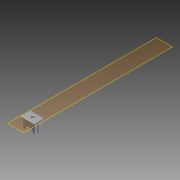
# Autodesk Inventor part: InternalKey
Saved by Autodesk Inventor 2012 (Build 160160000, 160)
## iProperties
Created: 2011-09-20
Part Number: InternalKey
Material: Default
Document SubType Name: Modeling
Designer: KuttaA
Density: 1 g/cm^3
Mass: 2.21175 g
Surface Area: 14.0837 cm^2
Volume: 2.21175 cm^3
Author: KuttaA
Autodesk Inventor part; units mm, degrees
ref_plane "YZ Plane" through (0, 0, 0) normal (1, 0, 0) x (0, 1, 0)
ref_plane "XZ Plane" through (0, 0, 0) normal (0, 1, 0) x (-1, 0, 0)
ref_plane "Work Plane8" through (7.15, 0.8, 25.4) normal (0, 1, 0) x (1, 0, 0)
sketch "Sketch21" plane through (7.15, 0.8, 25.4) normal (0, 1, 0) x (1, 0, 0)
  line L0 (-3, 3) -> (-24, 3)
  line L1 (-3, 197) -> (-3, 3)
  line L2 (-24, 197) -> (-3, 197)
  line L3 (-24, 3) -> (-24, 197)
  line L4 (-4.819988, 19.366667) -> (-3.319988, 19.366667)
  line L5 (-3.319988, 19.366667) -> (-3.319988, 16.033333)
  line L6 (-3.319988, 16.033333) -> (-4.819988, 16.033333)
  line L7 (-4.819988, 16.033333) -> (-4.819988, 12.7)
  line L8 (-4.819988, 12.7) -> (-22.180012, 12.7)
  line L9 (-22.180012, 12.7) -> (-22.180012, 16.033333)
  line L10 (-22.180012, 16.033333) -> (-23.680012, 16.033333)
  line L11 (-23.680012, 16.033333) -> (-23.680012, 19.366667)
  line L12 (-23.680012, 19.366667) -> (-22.180012, 19.366667)
  line L13 (-22.180012, 19.366667) -> (-22.180012, 22.7)
  line L14 (-22.180012, 22.7) -> (-4.819988, 22.7)
  line L15 (-4.819988, 22.7) -> (-4.819988, 19.366667)
  line L16 (-21.880012, 22.4) -> (-21.880012, 19.066667)
  line L17 (-21.880012, 19.066667) -> (-23.380012, 19.066667)
  line L18 (-23.380012, 19.066667) -> (-23.380012, 16.333333)
  line L19 (-23.380012, 16.333333) -> (-21.880012, 16.333333)
  line L20 (-21.880012, 16.333333) -> (-21.880012, 13)
  line L21 (-21.880012, 13) -> (-5.119988, 13)
  line L22 (-5.119988, 13) -> (-5.119988, 16.333333)
  line L23 (-5.119988, 16.333333) -> (-3.619988, 16.333333)
  line L24 (-3.619988, 16.333333) -> (-3.619988, 19.066667)
  line L25 (-3.619988, 19.066667) -> (-5.119988, 19.066667)
  line L26 (-5.119988, 19.066667) -> (-5.119988, 22.4)
  line L27 (-5.119988, 22.4) -> (-21.880012, 22.4)
  point P0 (-7.15, 25.4)
  dimension "d99" = 0.3
  dimension "d100" = 0.3
  dimension "d101" = 0.3
  dimension "d102" = 0.3
  dimension "d103" = 0.3
  dimension "d104" = 0.3
  dimension "d105" = 0.3
  dimension "d106" = 0.3
  dimension "d107" = 0.3
  dimension "d108" = 0.3
  dimension "d109" = 0.3
  dimension "d110" = 0.3
  constraints: 24 end point, 8 parallel, 2 collinear, 2 perpendicular
  measures "d99" distance between parallel lines of L14 L27
  measures "d100" distance between parallel lines of L15 L26
  measures "d101" distance between parallel lines of L4 L25
  measures "d102" distance between parallel lines of L5 L24
  measures "d103" distance between parallel lines of L6 L23
  measures "d104" distance between parallel lines of L7 L22
  measures "d105" distance between parallel lines of L8 L21
  measures "d106" distance between parallel lines of L9 L20
  measures "d107" distance between parallel lines of L10 L19
  measures "d108" distance between parallel lines of L11 L18
  measures "d109" distance between parallel lines of L12 L17
  measures "d110" distance between parallel lines of L13 L16
ref_plane "Work Plane9" through (-1.05, -12.7, 2.7) normal (0, 1, 0) x (0, 0, 1)
sketch "Sketch21 outline for Extrusion20" plane through (7.15, 0.8, 25.4) normal (0, 1, 0) x (1, 0, 0)
  line L0 (-5.119988, 22.4) -> (-21.880012, 22.4)
  line L1 (-5.119988, 19.066667) -> (-5.119988, 22.4)
  line L2 (-3.619988, 19.066667) -> (-5.119988, 19.066667)
  line L3 (-3.619988, 16.333333) -> (-3.619988, 19.066667)
  line L4 (-5.119988, 16.333333) -> (-3.619988, 16.333333)
  line L5 (-5.119988, 13) -> (-5.119988, 16.333333)
  line L6 (-21.880012, 13) -> (-5.119988, 13)
  line L7 (-21.880012, 16.333333) -> (-21.880012, 13)
  line L8 (-23.380012, 16.333333) -> (-21.880012, 16.333333)
  line L9 (-23.380012, 19.066667) -> (-23.380012, 16.333333)
  line L10 (-21.880012, 19.066667) -> (-23.380012, 19.066667)
  line L11 (-21.880012, 22.4) -> (-21.880012, 19.066667)
extrude "Extrusion20" add sketch "Sketch21 outline for Extrusion20" against normal up to surface (13.5 mm away)
sketch "Sketch22" plane through (-14.730012, 0.8, 12.4) normal (0, 0, 1) x (1, 0, 0)
  circle A0 centre (8.380012, -13.5) radius 5 construction
  arc A1 (3.080012, -13.5) -> (13.680012, -13.5) centre (8.380012, -13.5) ccw
  arc A2 (13.680012, -13.5) -> (3.080012, -13.5) centre (8.380012, -13.5) ccw
  point P0 (14.730012, -0.8)
  constraints: 2 point on circle, 1 centre point, 1 concentric
sketch "Sketch22 outline for Extrusion21" plane through (-14.730012, 0.8, 12.4) normal (0, 0, 1) x (1, 0, 0)
  arc A0 (13.680012, -13.5) -> (3.080012, -13.5) centre (8.380012, -13.5) ccw
  arc A1 (3.080012, -13.5) -> (13.680012, -13.5) centre (8.380012, -13.5) ccw
extrude "Extrusion21" cut sketch "Sketch22 outline for Extrusion21" against normal through all
sketch "Sketch23" plane through (7.15, 0.8, 25.4) normal (0, 1, 0) x (1, 0, 0)
  line L0 (-21.880012, 22.4) -> (-21.880012, 19.066667)
  line L1 (-21.880012, 19.066667) -> (-23.380012, 19.066667)
  line L2 (-23.380012, 19.066667) -> (-23.380012, 16.333333)
  line L3 (-23.380012, 16.333333) -> (-21.880012, 16.333333)
  line L4 (-21.880012, 16.333333) -> (-21.880012, 13)
  line L5 (-21.880012, 13) -> (-5.119988, 13)
  line L6 (-5.119988, 13) -> (-5.119988, 16.333333)
  line L7 (-5.119988, 16.333333) -> (-3.619988, 16.333333)
  line L8 (-3.619988, 16.333333) -> (-3.619988, 19.066667)
  line L9 (-3.619988, 19.066667) -> (-5.119988, 19.066667)
  line L10 (-5.119988, 19.066667) -> (-5.119988, 22.4)
  line L11 (-5.119988, 22.4) -> (-21.880012, 22.4)
  line L12 (-24, 3) -> (-24, 197)
  line L13 (-3, 197) -> (-3, 3)
  line L14 (-23.680012, 24.9) -> (-3.319988, 24.9)
  line L15 (-3.319988, 24.9) -> (-3.319988, 10.5)
  line L16 (-3.319988, 10.5) -> (-23.680012, 10.5)
  line L17 (-23.680012, 10.5) -> (-23.680012, 24.9)
  point P0 (-7.15, 25.4)
  dimension "d115" = 2.5
  dimension "d116" = 2.5
  dimension "d117" = 0.3
  dimension "d118" = 0.3
  constraints: 8 end point, 2 parallel, 1 horizontal, 1 perpendicular
  measures "d115" distance between parallel lines of L14 L11
  measures "d116" distance between parallel lines of L16 L5
  measures "d117" distance between parallel lines of L2 L17
  measures "d118" distance between parallel lines of L15 L8
sketch "Sketch23 outline for Extrusion22" plane through (7.15, 0.8, 25.4) normal (0, 1, 0) x (1, 0, 0)
  line L0 (-23.680012, 24.9) -> (-3.319988, 24.9)
  line L1 (-3.319988, 24.9) -> (-3.319988, 10.5)
  line L2 (-3.319988, 10.5) -> (-23.680012, 10.5)
  line L3 (-23.680012, 10.5) -> (-23.680012, 24.9)
extrude "Extrusion22" add sketch "Sketch23 outline for Extrusion22" along normal blind 1.5
sketch "Sketch24" plane through (-16.530012, 0.8, 14.9) normal (0, 0, 1) x (1, 0, 0)
  line L0 (20.360025, 1.5) -> (0, 1.5)
  line L1 (0, 0) -> (0, 1.5)
  line L2 (20.360025, 0) -> (0, 0)
  line L3 (20.360025, 0) -> (20.360025, 1.5)
  line L4 (6.786675, 0) -> (13.57335, 0)
  line L5 (13.57335, 0) -> (13.57335, 0.75)
  line L6 (13.57335, 0.75) -> (6.786675, 0.75)
  line L7 (6.786675, 0.75) -> (6.786675, 0)
  point P0 (16.530012, -0.8)
  dimension "d121" = 20.36002
  dimension "d122" = 6.78667
  dimension "d123" = 6.78667
  dimension "d124" = 0.75
  dimension "d125" = 1.5
  constraints: 8 end point, 2 parallel, 1 horizontal, 1 perpendicular, 1 point on line
  measures "d121" distance of L2.start L1.start
  measures "d122" distance of L5.end L6.end
  measures "d123" distance between parallel lines of L3 L5
  measures "d124" distance between parallel lines of L2 L6
  measures "d125" distance between parallel lines of L2 L0
sketch "Sketch24 outline for Extrusion23" plane through (-16.530012, 0.8, 14.9) normal (0, 0, 1) x (1, 0, 0)
  line L0 (6.786675, 0.75) -> (6.786675, 0)
  line L1 (13.57335, 0.75) -> (6.786675, 0.75)
  line L2 (13.57335, 0) -> (13.57335, 0.75)
  line L3 (6.786675, 0) -> (13.57335, 0)
extrude "Extrusion23" cut sketch "Sketch24 outline for Extrusion23" against normal blind 1.5
sketch "Sketch25" plane through (3.830012, 0.8, 0.5) normal (0, 0, -1) x (-1, 0, 0)
  line L0 (6.786675, 0.75) -> (6.786675, 0)
  line L1 (13.57335, 0.75) -> (6.786675, 0.75)
  line L2 (13.57335, 0) -> (13.57335, 0.75)
  line L3 (20.360025, 0) -> (0, 0)
  point P0 (3.830012, -0.8)
fillet "Fillet13" radius 2 3 edges at (-9.7433, 1.55, 14.15) (-2.9567, 1.55, 14.15) (-6.35, 1.55, 13.4)
sketch "Sketch25 outline for Extrusion24" plane through (3.830012, 0.8, 0.5) normal (0, 0, -1) x (-1, 0, 0)
  line L0 (13.57335, 0.75) -> (6.786675, 0.75)
  line L1 (13.57335, 0) -> (13.57335, 0.75)
  line L2 (6.786675, 0) -> (13.57335, 0)
  line L3 (6.786675, 0.75) -> (6.786675, 0)
extrude "Extrusion24" cut sketch "Sketch25 outline for Extrusion24" against normal blind 1.5
fillet "Fillet14" radius 2 3 edges at (-2.9567, 1.55, 1.25) (-9.7433, 1.55, 1.25) (-6.35, 1.55, 2)
fillet "Fillet15" radius 1 8 edges at (-6.35, 2.3, 0.5) (3.83, 2.3, 7.7) (-6.35, 2.3, 14.9) (-16.53, 2.3, 7.7) (3.83, 1.55, 0.5) (3.83, 1.55, 14.9) (-16.53, 1.55, 0.5) (-16.53, 1.55, 14.9)
sketch "Sketch26" plane through (-16.230012, -12.7, 9.066667) normal (0, -1, 0) x (1, 0, 0)
  line L0 (4.580012, -6.066667) -> (4.580012, 3.333333)
  line L1 (4.580012, 3.333333) -> (1.5, 3.333333)
  line L2 (1.5, 3.333333) -> (1.5, 0)
  line L3 (1.5, 0) -> (0, 0)
  line L4 (0, 0) -> (0, -2.733333)
  line L5 (0, -2.733333) -> (1.5, -2.733333)
  line L6 (1.5, -2.733333) -> (1.5, -6.066667)
  line L7 (1.5, -6.066667) -> (4.580012, -6.066667)
  line L8 (15.180012, 3.333333) -> (15.180012, -6.066667)
  line L9 (15.180012, -6.066667) -> (18.260025, -6.066667)
  line L10 (18.260025, -6.066667) -> (18.260025, -2.733333)
  line L11 (18.260025, -2.733333) -> (19.760025, -2.733333)
  line L12 (19.760025, -2.733333) -> (19.760025, 0)
  line L13 (19.760025, 0) -> (18.260025, 0)
  line L14 (18.260025, 0) -> (18.260025, 3.333333)
  line L15 (18.260025, 3.333333) -> (15.180012, 3.333333)
  point P0 (16.230012, -9.066667)
sketch "Sketch26 outline for Extrusion25" plane through (-16.230012, -12.7, 9.066667) normal (0, -1, 0) x (1, 0, 0)
  line L0 (1.5, -6.066667) -> (4.580012, -6.066667)
  line L1 (1.5, -2.733333) -> (1.5, -6.066667)
  line L2 (0, -2.733333) -> (1.5, -2.733333)
  line L3 (0, 0) -> (0, -2.733333)
  line L4 (1.5, 0) -> (0, 0)
  line L5 (1.5, 3.333333) -> (1.5, 0)
  line L6 (4.580012, 3.333333) -> (1.5, 3.333333)
  line L7 (4.580012, -6.066667) -> (4.580012, 3.333333)
  line L8 (18.260025, 3.333333) -> (15.180012, 3.333333)
  line L9 (18.260025, 0) -> (18.260025, 3.333333)
  line L10 (19.760025, 0) -> (18.260025, 0)
  line L11 (19.760025, -2.733333) -> (19.760025, 0)
  line L12 (18.260025, -2.733333) -> (19.760025, -2.733333)
  line L13 (18.260025, -6.066667) -> (18.260025, -2.733333)
  line L14 (15.180012, -6.066667) -> (18.260025, -6.066667)
  line L15 (15.180012, 3.333333) -> (15.180012, -6.066667)
extrude "Extrusion25" cut sketch "Sketch26 outline for Extrusion25" against normal blind 0.15
sketch "Sketch27" plane through (7.15, 0.8, 25.4) normal (0, -1, 0) x (1, 0, 0)
  line L0 (-3.619988, -16.333333) -> (-3.619988, -19.066667)
  line L1 (-3.619988, -19.066667) -> (-5.119988, -19.066667)
  line L2 (-5.119988, -19.066667) -> (-5.119988, -22.4)
  line L3 (-5.119988, -22.4) -> (-21.880012, -22.4)
  line L4 (-21.880012, -22.4) -> (-21.880012, -19.066667)
  line L5 (-21.880012, -19.066667) -> (-23.380012, -19.066667)
  line L6 (-23.380012, -19.066667) -> (-23.380012, -16.333333)
  line L7 (-23.380012, -16.333333) -> (-21.880012, -16.333333)
  line L8 (-21.880012, -16.333333) -> (-21.880012, -13)
  line L9 (-21.880012, -13) -> (-5.119988, -13)
  line L10 (-5.119988, -13) -> (-5.119988, -16.333333)
  line L11 (-5.119988, -16.333333) -> (-3.619988, -16.333333)
  arc A0 (-22.680012, -10.5) -> (-23.680012, -11.5) centre (-22.680012, -11.5) ccw
  line L12 (-23.680012, -11.5) -> (-23.680012, -23.9)
  arc A1 (-23.680012, -23.9) -> (-22.680012, -24.9) centre (-22.680012, -23.9) ccw
  line L13 (-22.680012, -24.9) -> (-16.893337, -24.9)
  line L14 (-16.893337, -24.9) -> (-16.893337, -23.4)
  line L15 (-16.893337, -23.4) -> (-10.106663, -23.4)
  line L16 (-10.106663, -23.4) -> (-10.106663, -24.9)
  line L17 (-10.106663, -24.9) -> (-4.319988, -24.9)
  arc A2 (-4.319988, -24.9) -> (-3.319988, -23.9) centre (-4.319988, -23.9) ccw
  line L18 (-3.319988, -23.9) -> (-3.319988, -11.5)
  arc A3 (-3.319988, -11.5) -> (-4.319988, -10.5) centre (-4.319988, -11.5) ccw
  line L19 (-4.319988, -10.5) -> (-10.106663, -10.5)
  line L20 (-10.106663, -10.5) -> (-10.106663, -12)
  line L21 (-10.106663, -12) -> (-16.893337, -12)
  line L22 (-16.893337, -12) -> (-16.893337, -10.5)
  line L23 (-16.893337, -10.5) -> (-22.680012, -10.5)
  point P0 (-7.15, -25.4)
sketch "Sketch27 outline for Extrusion26" plane through (7.15, 0.8, 25.4) normal (0, -1, 0) x (1, 0, 0)
  line L0 (-16.893337, -10.5) -> (-22.680012, -10.5)
  line L1 (-16.893337, -12) -> (-16.893337, -10.5)
  arc A0 (-22.680012, -10.5) -> (-23.680012, -11.5) centre (-22.680012, -11.5) ccw
  line L2 (-10.106663, -12) -> (-16.893337, -12)
  line L3 (-23.680012, -11.5) -> (-23.680012, -23.9)
  line L4 (-10.106663, -10.5) -> (-10.106663, -12)
  arc A1 (-23.680012, -23.9) -> (-22.680012, -24.9) centre (-22.680012, -23.9) ccw
  line L5 (-4.319988, -10.5) -> (-10.106663, -10.5)
  line L6 (-22.680012, -24.9) -> (-16.893337, -24.9)
  arc A2 (-3.319988, -11.5) -> (-4.319988, -10.5) centre (-4.319988, -11.5) ccw
  line L7 (-16.893337, -24.9) -> (-16.893337, -23.4)
  line L8 (-3.319988, -23.9) -> (-3.319988, -11.5)
  line L9 (-16.893337, -23.4) -> (-10.106663, -23.4)
  arc A3 (-4.319988, -24.9) -> (-3.319988, -23.9) centre (-4.319988, -23.9) ccw
  line L10 (-10.106663, -23.4) -> (-10.106663, -24.9)
  line L11 (-10.106663, -24.9) -> (-4.319988, -24.9)
  line L12 (-5.119988, -16.333333) -> (-3.619988, -16.333333)
  line L13 (-5.119988, -13) -> (-5.119988, -16.333333)
  line L14 (-21.880012, -13) -> (-5.119988, -13)
  line L15 (-21.880012, -16.333333) -> (-21.880012, -13)
  line L16 (-23.380012, -16.333333) -> (-21.880012, -16.333333)
  line L17 (-23.380012, -19.066667) -> (-23.380012, -16.333333)
  line L18 (-21.880012, -19.066667) -> (-23.380012, -19.066667)
  line L19 (-21.880012, -22.4) -> (-21.880012, -19.066667)
  line L20 (-5.119988, -22.4) -> (-21.880012, -22.4)
  line L21 (-5.119988, -19.066667) -> (-5.119988, -22.4)
  line L22 (-3.619988, -19.066667) -> (-5.119988, -19.066667)
  line L23 (-3.619988, -16.333333) -> (-3.619988, -19.066667)
extrude "Extrusion26" cut sketch "Sketch27 outline for Extrusion26" against normal blind 0.15
sketch "Sketch28" plane through (7.15, 2.3, 25.4) normal (0, 1, 0) x (1, 0, 0)
  circle A0 centre (-13.5, 17.7) radius 2
  point P0 (-7.15, 25.4)
  constraints: 1 centre point, 2 other
sketch "Sketch28 outline for Extrusion27" plane through (7.15, 2.3, 25.4) normal (0, 1, 0) x (1, 0, 0)
  circle A0 centre (-13.5, 17.7) radius 2
extrude "Extrusion27" cut sketch "Sketch28 outline for Extrusion27" against normal blind 5
equation "\"d100\" = d99"
equation "\"d101\" = d99"
equation "\"d102\" = d101"
equation "\"d103\" = d102"
equation "\"d104\" = d102"
equation "\"d105\" = d104"
equation "\"d106\" = d105"
equation "\"d107\" = d106"
equation "\"d108\" = d106"
equation "\"d109\" = d107"
equation "\"d110\" = d109"
equation "\"d116\" = d115"
equation "\"d118\" = d117"
equation "\"d122\" = 0.333333 * d121"
equation "\"d123\" = d122"
equation "\"d124\" = 0.5 * d125"
body "Solid5"
